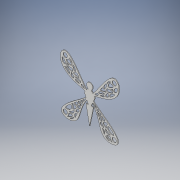
# Autodesk Inventor part: Dragonfly_PCB
Saved by Autodesk Inventor 2019 (Build 230136000, 136)
## iProperties
Created: 2019-03-17
Part Number: Dragonfly_PCB
Material: Generic
Document SubType Name: Modeling
Designer: cutla
Density: 1 g/cm^3
Appearance: Default
Author: cutla
Autodesk Inventor part; units mm, degrees
ref_plane "YZ Plane" through (0, 0, 0) normal (1, 0, 0) x (0, 1, 0)
ref_plane "XZ Plane" through (0, 0, 0) normal (0, 1, 0) x (-1, 0, 0)
ref_plane "XY Plane" through (0, 0, 0) normal (0, 0, 1) x (1, 0, 0)
sketch "Sketch1" plane through (0, 0, 0) normal (0, 0, 1) x (1, 0, 0)
  circle A0 centre (0, 16.1725) radius 5
  line L0 (-50, 50) -> (50, 50) construction
  line L1 (50, 50) -> (50, -50) construction
  line L2 (50, -50) -> (-50, -50) construction
  line L3 (-50, -50) -> (-50, 50) construction
  line L4 (-3.4999, 10.6039) -> (-2.6514, 10.6039)
  line L5 (0, 50) -> (0, -50) construction
  line L6 (-3.5, 10.6039) -> (-8.6386, 3.3725)
  line L7 (-8.6386, 3.3725) -> (-2.5, -10.2779)
  line L8 (2.2173, -10.2779) -> (2.4999, -10.2779)
  line L9 (-6, -11.0793) -> (-0.1613, -40.5057)
  line L10 (-0.1613, -40.5057) -> (6, -11.0793)
  circle A1 centre (-40, 40) radius 23 construction
  circle A2 centre (-40, 40) radius 3.5
  circle A3 centre (-40, 40) radius 6.5 construction
  circle A4 centre (40, 40) radius 23 construction
  circle A5 centre (40, 40) radius 3.5
  circle A6 centre (40, 40) radius 6.5 construction
  line L11 (-50, 0) -> (50, 0) construction
  circle A7 centre (-40, -40) radius 23 construction
  circle A8 centre (-40, -40) radius 3.5
  circle A9 centre (-40, -40) radius 6.5 construction
  circle A10 centre (40, -40) radius 23 construction
  circle A11 centre (40, -40) radius 6.5 construction
  circle A12 centre (40, -40) radius 3.5
  line L12 (-40, 40) -> (40, -40) construction
  line L13 (40, 40) -> (-40, -40) construction
  spline S0 degree 4 poles (-7.4222, 5.0843) (-12.8668, 9.132) (-70.5582, 8.2428) (-44.5421, 80.9884) (-22.7349, 29.3004) (-5.2813, 8.0972) knots 0 0 0 0 0 0.479158 1 1 1 1 1
  spline S1 degree 4 poles (-6, -2.495) (-20.1858, -15.9699) (-90.0237, -50.8952) (-1.0731, -60.254) (-21.894, -29.1199) (-4.4831, -5.8681) knots 0 0 0 0 0 0.512159 1 1 1 1 1
  line L14 (3.5, 10.6039) -> (8.6386, 3.3726)
  line L15 (8.6386, 3.3725) -> (2.5, -10.2779)
  spline S2 degree 4 poles (7.4222, 5.0843) (12.8668, 9.132) (70.5582, 8.2428) (44.5421, 80.9884) (22.7349, 29.3004) (5.2813, 8.0972) knots 0 0 0 0 0 0.479158 1 1 1 1 1
  spline S3 degree 4 poles (6, -2.495) (20.1858, -15.9699) (90.0237, -50.8952) (1.0731, -60.254) (21.894, -29.1199) (4.4831, -5.8681) knots 0 0 0 0 0 0.512159 1 1 1 1 1
  line L16 (-2.1572, -10.5653) -> (-3.3324, -11.0793)
  line L17 (2.1572, -10.5653) -> (3.3324, -11.0793)
  line L18 (-3.0807, 12.2343) -> (-2.6513, 10.6041)
  line L19 (3.0807, 12.2343) -> (2.6513, 10.6041)
  arc A13 (-3.4999, 10.6039) -> (-3.5, 10.6039) centre (-3.4999, 10.6038) ccw
  arc A14 (-2.6514, 10.6039) -> (-2.6513, 10.6041) centre (-2.6514, 10.604) ccw
  line L20 (2.6514, 10.6039) -> (3.4999, 10.6039)
  arc A15 (2.6513, 10.6041) -> (2.6514, 10.6039) centre (2.6514, 10.604) ccw
  arc A16 (3.5, 10.6039) -> (3.4999, 10.6039) centre (3.4999, 10.6038) ccw
  arc A17 (8.6386, 3.3725) -> (8.6386, 3.3726) centre (8.6385, 3.3725) ccw
  arc A18 (1.5005, -10.2779) -> (1.5004, -10.2781) centre (1.5005, -10.278) ccw
  line L21 (-2.5, -10.2779) -> (-2.2173, -10.2779)
  line L22 (-6, -11.0793) -> (-3.3324, -11.0793)
  line L23 (3.3324, -11.0793) -> (6, -11.0793)
  arc A19 (-3.3324, -11.0793) -> (-3.3324, -11.0793) centre (-3.3324, -11.0792) ccw
  arc A20 (-1.5004, -10.2781) -> (-1.5005, -10.2779) centre (-1.5005, -10.278) ccw
  arc A21 (1.5005, -10.2779) -> (1.5004, -10.2781) centre (1.5005, -10.278) ccw
  arc A22 (2.4999, -10.2779) -> (2.5, -10.2779) centre (2.4999, -10.2778) ccw
  arc A23 (3.3324, -11.0793) -> (3.3324, -11.0793) centre (3.3324, -11.0792) ccw
  line L24 (-3.0807, 12.2343) -> (3.0807, 12.2343)
  arc A24 (-2.1572, -10.5653) -> (-2.2173, -10.2779) centre (-2.2173, -10.4279) ccw
  arc A25 (2.2173, -10.2779) -> (2.1572, -10.5653) centre (2.2173, -10.4279) ccw
  point P0 (0, 0)
  point P1 (-3.5, 10.6039)
  point P2 (3.5, 10.6039)
  point P3 (2.5, -10.2779)
  point P4 (-3.5, 10.6039)
  point P5 (0, 25.4731)
  point P6 (0, 0)
  point P7 (0, 2.9442)
  point P8 (-47.4996, 31.0772)
  point P9 (-44.5962, 44.5962)
  point P10 (-36.5, 45.4772)
  point P11 (-30.415, 12.5972)
  point P12 (-44.5962, -35.4038)
  point P13 (-44.5962, -44.5962)
  point P14 (-32.1189, -47.8681)
  point P15 (-20.478, -41.302)
  point P16 (3.5, 10.6039)
  point P17 (8.6386, 3.3725)
  point P18 (47.4996, 31.0772)
  point P19 (44.5962, 44.5962)
  point P20 (36.5, 45.4772)
  point P21 (30.415, 12.5972)
  point P22 (44.5962, -35.4038)
  point P23 (44.5962, -44.5962)
  point P24 (32.1189, -47.8681)
  point P25 (20.478, -41.302)
  point P26 (0, -11.0793)
  point P27 (0, 0)
  point P28 (-1.5, -10.2779)
  point P29 (-3.3324, -11.0793)
  point P30 (1.5, -10.2779)
  point P31 (-2.6512, 10.6039)
  point P32 (2.6512, 10.6039)
  point P33 (3.3324, -11.0793)
  dimension "d0" = 10
  dimension "d1" = 100
  dimension "d2" = 100
  dimension "d3" = 7
  dimension "d5" = 12
  dimension "d6" = 30
  dimension "d7" = 5
  dimension "d8" = 46
  dimension "d9" = 40
  dimension "d10" = 40
  dimension "d11" = 7
  dimension "d12" = 3
  dimension "d13" = 2
  dimension "d14" = 0.0001
  dimension "d15" = 0.0001
  dimension "d16" = 0.0001
  dimension "d24" = 0.15
  constraints: 50 end point, 38 point on line, 30 point on circle, 26 tangent, 25 centre point, 24 symmetric about line, 9 equal radius, 8 horizontal, 6 midpoint, 4 coincident, 4 vertical alignment, 2 parallel, 2 perpendicular, 1 horizontal alignment, 36 other
  measures "d1" distance of L1.end L2.end
  measures "d2" distance of L0.end L1.end
  measures "d3" distance of point (-3.5, 10.604) point (3.5, 10.604)
  measures "d5" distance of L9.start L10.end
  measures "d6" distance of L9.start L9.end
  measures "d7" distance of L7.end point (2.5, -10.278)
  measures "d8" diameter of A1
  measures "d9" distance from line of L5 A1.centre
  measures "d10" horizontal distance of point (0, 0) A1.centre
  measures "d11" diameter of A2
  measures "d12" radial gap between concentric circles of A2 A3
  measures "d13" distance of point (-1.5, -10.278) point (-3.332, -11.079)
  measures "d14" radius of A13
  measures "d15" radius of A15
  measures "d16" radius of A19
  measures "d24" radius of A24
extrude "Extrusion2" add sketch "Sketch1" along normal blind 1 contours A0 L24 | A23 | A19 | A13 | L24 A0 | A0 L19 L20 L14 L15 L8 A25 L17 L23 L10 L9 L22 L16 A24 L21 L7 L6 L4 L18 | L6 S0 | S2 L14 | L7 S1 | S3 L15 | A18 | A20
sketch "Sketch2" plane through (0, 0, 1) normal (0, 0, 1) x (1, 0, 0)
  circle A0 centre (40, 40) radius 3.5 projected
  circle A1 centre (40, -40) radius 3.5 projected
  circle A2 centre (-40, -40) radius 3.5 projected
  circle A3 centre (-40, 40) radius 3.5 projected
  line L0 (-3.0807, 12.2343) -> (-2.6513, 10.6041) projected
  arc A4 (-2.6514, 10.6039) -> (-2.6513, 10.6041) centre (-2.6514, 10.604) ccw projected
  line L1 (-2.6514, 10.6039) -> (-3.4999, 10.6039) projected
  arc A5 (-3.4999, 10.6039) -> (-3.5, 10.6039) centre (-3.4999, 10.6038) ccw projected
  line L2 (-3.5, 10.6039) -> (-5.2813, 8.0972) projected
  line L3 (-7.4222, 5.0843) -> (-8.6386, 3.3725) projected
  line L4 (-8.6386, 3.3725) -> (-6, -2.495) projected
  line L5 (-4.4831, -5.8681) -> (-2.5, -10.2779) projected
  line L6 (-2.5, -10.2779) -> (-2.2173, -10.2779) projected
  line L7 (-2.1572, -10.5653) -> (-3.3324, -11.0793) projected
  arc A6 (-3.3324, -11.0793) -> (-3.3324, -11.0793) centre (-3.3324, -11.0792) ccw projected
  line L8 (-3.3324, -11.0793) -> (-6, -11.0793) projected
  line L9 (-6, -11.0793) -> (-0.1613, -40.5057) projected
  line L10 (-0.1613, -40.5057) -> (6, -11.0793) projected
  line L11 (6, -11.0793) -> (3.3324, -11.0793) projected
  arc A7 (3.3324, -11.0793) -> (3.3324, -11.0793) centre (3.3324, -11.0792) ccw projected
  line L12 (3.3324, -11.0793) -> (2.1572, -10.5653) projected
  line L13 (2.2173, -10.2779) -> (2.4999, -10.2779) projected
  arc A8 (2.4999, -10.2779) -> (2.5, -10.2779) centre (2.4999, -10.2778) ccw projected
  line L14 (2.5, -10.2779) -> (4.4831, -5.8681) projected
  line L15 (6, -2.495) -> (8.6386, 3.3725) projected
  arc A9 (8.6386, 3.3725) -> (8.6386, 3.3726) centre (8.6385, 3.3725) ccw projected
  line L16 (8.6386, 3.3726) -> (7.4222, 5.0843) projected
  line L17 (5.2813, 8.0972) -> (3.5, 10.6039) projected
  arc A10 (3.5, 10.6039) -> (3.4999, 10.6039) centre (3.4999, 10.6038) ccw projected
  line L18 (3.4999, 10.6039) -> (2.6514, 10.6039) projected
  arc A11 (2.6513, 10.6041) -> (2.6514, 10.6039) centre (2.6514, 10.604) ccw projected
  line L19 (2.6513, 10.6041) -> (3.0807, 12.2343) projected
  arc A12 (3.0807, 12.2343) -> (-3.0807, 12.2343) centre (0, 16.1725) ccw projected
  spline S0 degree 5 poles (-44.3024, 35.4148) (-45.0994, 35.5233) (-45.8132, 34.3852) (-44.5065, 29.4541) (-43.5224, 26.3569) (-36.151, 26.1839) (-40.7739, 33.1916) (-43.3141, 35.2801) (-44.3024, 35.4148) knots 0 0 0 0 0 0 0.267852 0.467852 0.667852 1 1 1 1 1 1
  spline S1 degree 5 poles (-40.9057, 24.138) (-41.3791, 23.8252) (-40.5305, 22.4203) (-34.97, 18.6489) (-32.8952, 14.2131) (-29.9643, 20.7538) (-37.6368, 24.0325) (-40.3884, 24.4797) (-40.9057, 24.138) knots 0 0 0 0 0 0 0.286709 0.486709 0.686709 1 1 1 1 1 1
  spline S2 degree 5 poles (-35.4207, 23.9165) (-33.7431, 23.259) (-30.5035, 22.0511) (-26.908, 20.6903) (-24.0215, 30.7808) (-39.446, 25.8859) (-39.0589, 25.3943) (-36.9204, 24.5043) (-35.4207, 23.9165) knots 0 0 0 0 0 0 0.31679 0.51679 0.71679 1 1 1 1 1 1
  spline S3 degree 5 poles (-38.2164, 33.6068) (-38.4732, 34.7959) (-37.0442, 36.9005) (-30.4365, 38.8601) (-30.2842, 28.8387) (-28.4964, 29.5351) (-35.694, 30.5745) (-37.9609, 32.4241) (-38.2164, 33.6068) knots 0 0 0 0 0 0 0.300806 0.500806 0.700806 1 1 1 1 1 1
  spline S4 degree 5 poles (-37.7279, 30.3885) (-37.4976, 30.6871) (-36.795, 30.6092) (-34.7596, 28.9094) (-31.9567, 29.1222) (-38.1366, 27.3933) (-37.545, 26.8348) (-37.9995, 29.2023) (-37.9352, 30.1199) (-37.7279, 30.3885) knots 0 0 0 0 0 0 0.257793 0.412829 0.612829 0.768046 1 1 1 1 1 1
  spline S5 degree 5 poles (-29.5965, 20.8413) (-30.028, 21.0016) (-30.3312, 20.3769) (-29.4621, 17.0894) (-34.8392, 16.5928) (-21.6573, 10.7431) (-26.8093, 18.2659) (-28.9115, 20.5868) (-29.5965, 20.8413) knots 0 0 0 0 0 0 0.231873 0.431873 0.631873 1 1 1 1 1 1
  spline S6 degree 5 poles (-21.2933, 24.138) (-22.1912, 24.1136) (-24.1767, 23.296) (-28.4063, 20.5075) (-28.5904, 21.6776) (-12.6977, 16.5147) (-18.9526, 20.044) (-19.372, 23.4263) (-20.3779, 24.1629) (-21.2933, 24.138) knots 0 0 0 0 0 0 0.240115 0.403809 0.603809 0.755207 1 1 1 1 1 1
  spline S7 degree 5 poles (-23.6063, 17.5202) (-22.4674, 17.6083) (-19.6677, 17.7476) (-15.5206, 18.27) (-8.8964, 8.6854) (-23.9906, 16.981) (-25.349, 17.3364) (-24.46, 17.4541) (-23.6063, 17.5202) knots 0 0 0 0 0 0 0.342928 0.542928 0.742928 1 1 1 1 1 1
  spline S8 degree 5 poles (-22.8794, 14.1718) (-22.1093, 14.3621) (-20.5323, 14.072) (-18.6608, 12.0753) (-11.8654, 10.6615) (-24.2751, 11.1259) (-24.4556, 13.2266) (-23.5584, 14.0041) (-22.8794, 14.1718) knots 0 0 0 0 0 0 0.31884 0.51884 0.71884 1 1 1 1 1 1
  spline S9 degree 5 poles (-12.437, 12.2343) (-11.4678, 12.1009) (-9.6497, 10.9625) (-7.7008, 7.3802) (-7.7483, 8.7391) (-15.1459, 8.7266) (-14.7079, 11.7278) (-13.3583, 12.3611) (-12.437, 12.2343) knots 0 0 0 0 0 0 0.307615 0.507615 0.707615 1 1 1 1 1 1
  spline S10 degree 5 poles (-26.7763, 32.7115) (-26.2605, 32.367) (-25.2409, 31.2314) (-23.9711, 29.2562) (-22.0326, 28.1003) (-24.0441, 19.7801) (-28.4582, 31.1538) (-28.0163, 33.138) (-27.2677, 33.0398) (-26.7763, 32.7115) knots 0 0 0 0 0 0 0.235048 0.414891 0.614891 0.776086 1 1 1 1 1 1
  spline S11 degree 5 poles (-33.5613, 39.3254) (-33.0247, 39.4673) (-31.3289, 38.8651) (-27.3729, 34.9291) (-27.8955, 31.1209) (-31.3505, 38.4233) (-33.3068, 37.2083) (-34.1331, 38.6944) (-33.9123, 39.2325) (-33.5613, 39.3254) knots 0 0 0 0 0 0 0.293287 0.471191 0.671191 0.808125 1 1 1 1 1 1
  line L20 (0, 83.4672) -> (0, -77.3956) construction
  line L21 (-100, 0) -> (100, 0) construction
  spline S12 degree 5 poles (-39.2981, -34.2723) (-39.9524, -33.5365) (-39.0724, -31.2196) (-32.5116, -26.1597) (-30.2015, -22.1531) (-26.383, -31.7521) (-35.2925, -35.1565) (-38.6056, -35.0512) (-39.2981, -34.2723) knots 0 0 0 0 0 0 0.291485 0.491485 0.691485 1 1 1 1 1 1
  spline S13 degree 5 poles (-36.5, -44.8815) (-36.4507, -44.5828) (-35.4911, -43.4851) (-32.644, -40.5677) (-38.0691, -38.4909) (-23.0925, -37.7062) (-29.217, -42.1937) (-35.4081, -45.019) (-36.561, -45.2506) (-36.5, -44.8815) knots 0 0 0 0 0 0 0.213907 0.370528 0.570528 0.735669 1 1 1 1 1 1
  spline S14 degree 5 poles (-32.0039, -45.3695) (-31.8744, -45.6106) (-30.4318, -45.569) (-25.6943, -44.229) (-25.7935, -37.9612) (-26.8264, -42.3738) (-31.1459, -44.3025) (-32.1316, -45.1319) (-32.0039, -45.3695) knots 0 0 0 0 0 0 0.302166 0.502166 0.702166 1 1 1 1 1 1
  spline S15 degree 5 poles (-23.7965, -40) (-23.4775, -39.8625) (-22.9484, -38.6253) (-21.9445, -34.3415) (-17.0929, -31.1562) (-25.8468, -34.6171) (-25.1819, -37.6445) (-24.4279, -39.7279) (-24.0223, -40.0974) (-23.7965, -40) knots 0 0 0 0 0 0 0.272758 0.454007 0.654007 0.806897 1 1 1 1 1 1
  spline S16 degree 5 poles (-33.5613, -36.2711) (-33.4269, -36.7872) (-31.3838, -37.6032) (-24.4371, -38.1393) (-25.5572, -25.7037) (-25.9287, -34.0707) (-32.1902, -34.9016) (-33.6909, -35.7733) (-33.5613, -36.2711) knots 0 0 0 0 0 0 0.305417 0.505417 0.705417 1 1 1 1 1 1
  spline S17 degree 5 poles (-29.099, -22.9229) (-29.0937, -23.4948) (-28.0891, -24.8398) (-24.9737, -27.5316) (-32.4079, -32.1747) (-17.9133, -26.873) (-22.652, -22.0668) (-28.0304, -21.7022) (-29.1046, -22.3167) (-29.099, -22.9229) knots 0 0 0 0 0 0 0.229729 0.394709 0.594709 0.756471 1 1 1 1 1 1
  spline S18 degree 5 poles (-22.3856, -29.8406) (-21.7098, -28.8001) (-20.283, -26.4225) (-18.686, -22.6054) (-13.3004, -31.1371) (-23.325, -31.1181) (-23.5991, -31.589) (-22.9093, -30.647) (-22.3856, -29.8406) knots 0 0 0 0 0 0 0.338056 0.538056 0.738056 1 1 1 1 1 1
  spline S19 degree 5 poles (-25.0368, -20.0903) (-24.9262, -19.1243) (-23.0566, -17.2684) (-16.6088, -15.1482) (-21.8108, -18.0869) (-18.3297, -22.5789) (-23.8077, -22.2725) (-25.1397, -20.99) (-25.0368, -20.0903) knots 0 0 0 0 0 0 0.310671 0.510671 0.710671 1 1 1 1 1 1
  spline S20 degree 5 poles (-20.0653, -23.3991) (-20.1731, -22.7136) (-19.3903, -21.1156) (-15.982, -18.0375) (-17.4847, -19.0811) (-15.059, -22.4523) (-14.2695, -23.7016) (-18.6971, -24.7249) (-19.9485, -24.1412) (-20.0653, -23.3991) knots 0 0 0 0 0 0 0.244633 0.392961 0.592961 0.735209 1 1 1 1 1 1
  spline S21 degree 5 poles (-14.9655, -19.8082) (-15.4817, -19.9871) (-16.0939, -19.275) (-15.7797, -15.6875) (-12.5142, -14.9164) (-11.1676, -13.0261) (-13.0637, -17.9918) (-14.3713, -19.6023) (-14.9655, -19.8082) knots 0 0 0 0 0 0 0.278933 0.478933 0.678933 1 1 1 1 1 1
  spline S22 degree 5 poles (-18.6073, -14.8706) (-18.6874, -15.4171) (-18.5034, -16.4284) (-17.5929, -17.9229) (-17.0852, -19.6506) (-16.7442, -14.6538) (-12.8723, -15.347) (-16.1809, -12.8202) (-18.0104, -13.4255) (-18.5213, -14.2838) (-18.6073, -14.8706) knots 0 0 0 0 0 0 0.195722 0.324759 0.489124 0.649281 0.789869 1 1 1 1 1 1
  spline S23 degree 5 poles (-14.8166, -12.0066) (-14.9241, -12.6125) (-14.4296, -13.5435) (-11.7527, -14.1587) (-9.7456, -11.9141) (-12.6682, -11.6578) (-11.7181, -9.6006) (-13.973, -10.5064) (-14.7175, -11.4477) (-14.8166, -12.0066) knots 0 0 0 0 0 0 0.258357 0.41044 0.61044 0.761675 1 1 1 1 1 1
  spline S24 degree 5 poles (-9.9348, -7.5375) (-10.6244, -8.0811) (-11.5814, -8.9066) (-11.9107, -9.696) (-9.5983, -11.7884) (-7.6983, -7.6612) (-4.6953, -3.5354) (-7.2011, -5.498) (-9.0229, -6.8188) (-9.9348, -7.5375) knots 0 0 0 0 0 0 0.209184 0.360069 0.560069 0.723374 1 1 1 1 1 1
  circle A13 centre (40, -40) radius 3.5
  circle A14 centre (40, 40) radius 3.5
  line L22 (7.4222, 5.0843) -> (8.6386, 3.3725)
  line L23 (8.6386, 3.3725) -> (6, -2.495)
  spline S25 degree 5 poles (44.3024, 35.4148) (45.0994, 35.5233) (45.8132, 34.3852) (44.5065, 29.4541) (43.5224, 26.3569) (36.151, 26.1839) (40.7739, 33.1916) (43.3141, 35.2801) (44.3024, 35.4148) knots 0 0 0 0 0 0 0.267852 0.467852 0.667852 1 1 1 1 1 1
  spline S26 degree 5 poles (40.9057, 24.138) (41.3791, 23.8252) (40.5305, 22.4203) (34.97, 18.6489) (32.8952, 14.2131) (29.9643, 20.7538) (37.6368, 24.0325) (40.3884, 24.4797) (40.9057, 24.138) knots 0 0 0 0 0 0 0.286709 0.486709 0.686709 1 1 1 1 1 1
  spline S27 degree 5 poles (35.4207, 23.9165) (33.7431, 23.259) (30.5035, 22.0511) (26.908, 20.6903) (24.0215, 30.7808) (39.446, 25.8859) (39.0589, 25.3943) (36.9204, 24.5043) (35.4207, 23.9165) knots 0 0 0 0 0 0 0.31679 0.51679 0.71679 1 1 1 1 1 1
  spline S28 degree 5 poles (38.2164, 33.6068) (38.4732, 34.7959) (37.0442, 36.9005) (30.4365, 38.8601) (30.2842, 28.8387) (28.4964, 29.5351) (35.694, 30.5745) (37.9609, 32.4241) (38.2164, 33.6068) knots 0 0 0 0 0 0 0.300806 0.500806 0.700806 1 1 1 1 1 1
  spline S29 degree 5 poles (37.7279, 30.3885) (37.4976, 30.6871) (36.795, 30.6092) (34.7596, 28.9094) (31.9567, 29.1222) (38.1366, 27.3933) (37.545, 26.8348) (37.9995, 29.2023) (37.9352, 30.1199) (37.7279, 30.3885) knots 0 0 0 0 0 0 0.257793 0.412829 0.612829 0.768046 1 1 1 1 1 1
  spline S30 degree 5 poles (29.5965, 20.8413) (30.028, 21.0016) (30.3312, 20.3769) (29.4621, 17.0894) (34.8392, 16.5928) (21.6573, 10.7431) (26.8093, 18.2659) (28.9115, 20.5868) (29.5965, 20.8413) knots 0 0 0 0 0 0 0.231873 0.431873 0.631873 1 1 1 1 1 1
  spline S31 degree 5 poles (21.2933, 24.138) (22.1912, 24.1136) (24.1767, 23.296) (28.4063, 20.5075) (28.5904, 21.6776) (12.6977, 16.5147) (18.9526, 20.044) (19.372, 23.4263) (20.3779, 24.1629) (21.2933, 24.138) knots 0 0 0 0 0 0 0.240115 0.403809 0.603809 0.755207 1 1 1 1 1 1
  spline S32 degree 5 poles (23.6063, 17.5202) (22.4674, 17.6083) (19.6677, 17.7476) (15.5206, 18.27) (8.8964, 8.6854) (23.9906, 16.981) (25.349, 17.3364) (24.46, 17.4541) (23.6063, 17.5202) knots 0 0 0 0 0 0 0.342928 0.542928 0.742928 1 1 1 1 1 1
  spline S33 degree 5 poles (22.8794, 14.1718) (22.1093, 14.3621) (20.5323, 14.072) (18.6608, 12.0753) (11.8654, 10.6615) (24.2751, 11.1259) (24.4556, 13.2266) (23.5584, 14.0041) (22.8794, 14.1718) knots 0 0 0 0 0 0 0.31884 0.51884 0.71884 1 1 1 1 1 1
  spline S34 degree 5 poles (12.437, 12.2343) (11.4678, 12.1009) (9.6497, 10.9625) (7.7008, 7.3802) (7.7483, 8.7391) (15.1459, 8.7266) (14.7079, 11.7278) (13.3583, 12.3611) (12.437, 12.2343) knots 0 0 0 0 0 0 0.307615 0.507615 0.707615 1 1 1 1 1 1
  spline S35 degree 5 poles (26.7763, 32.7115) (26.2605, 32.367) (25.2409, 31.2314) (23.9711, 29.2562) (22.0326, 28.1003) (24.0441, 19.7801) (28.4582, 31.1538) (28.0163, 33.138) (27.2677, 33.0398) (26.7763, 32.7115) knots 0 0 0 0 0 0 0.235048 0.414891 0.614891 0.776086 1 1 1 1 1 1
  spline S36 degree 5 poles (33.5613, 39.3254) (33.0247, 39.4673) (31.3289, 38.8651) (27.3729, 34.9291) (27.8955, 31.1209) (31.3505, 38.4233) (33.3068, 37.2083) (34.1331, 38.6944) (33.9123, 39.2325) (33.5613, 39.3254) knots 0 0 0 0 0 0 0.293287 0.471191 0.671191 0.808125 1 1 1 1 1 1
  spline S37 degree 5 poles (39.2981, -34.2723) (39.9524, -33.5365) (39.0724, -31.2196) (32.5116, -26.1597) (30.2015, -22.1531) (26.383, -31.7521) (35.2925, -35.1565) (38.6056, -35.0512) (39.2981, -34.2723) knots 0 0 0 0 0 0 0.291485 0.491485 0.691485 1 1 1 1 1 1
  spline S38 degree 5 poles (36.5, -44.8815) (36.4507, -44.5828) (35.4911, -43.4851) (32.644, -40.5677) (38.0691, -38.4909) (23.0925, -37.7062) (29.217, -42.1937) (35.4081, -45.019) (36.561, -45.2506) (36.5, -44.8815) knots 0 0 0 0 0 0 0.213907 0.370528 0.570528 0.735669 1 1 1 1 1 1
  spline S39 degree 5 poles (32.0039, -45.3695) (31.8744, -45.6106) (30.4318, -45.569) (25.6943, -44.229) (25.7935, -37.9612) (26.8264, -42.3738) (31.1459, -44.3025) (32.1316, -45.1319) (32.0039, -45.3695) knots 0 0 0 0 0 0 0.302166 0.502166 0.702166 1 1 1 1 1 1
  spline S40 degree 5 poles (23.7965, -40) (23.4775, -39.8625) (22.9484, -38.6253) (21.9445, -34.3415) (17.0929, -31.1562) (25.8468, -34.6171) (25.1819, -37.6445) (24.4279, -39.7279) (24.0223, -40.0974) (23.7965, -40) knots 0 0 0 0 0 0 0.272758 0.454007 0.654007 0.806897 1 1 1 1 1 1
  spline S41 degree 5 poles (33.5613, -36.2711) (33.4269, -36.7872) (31.3838, -37.6032) (24.4371, -38.1393) (25.5572, -25.7037) (25.9287, -34.0707) (32.1902, -34.9016) (33.6909, -35.7733) (33.5613, -36.2711) knots 0 0 0 0 0 0 0.305417 0.505417 0.705417 1 1 1 1 1 1
  spline S42 degree 5 poles (29.099, -22.9229) (29.0937, -23.4948) (28.0891, -24.8398) (24.9737, -27.5316) (32.4079, -32.1747) (17.9133, -26.873) (22.652, -22.0668) (28.0304, -21.7022) (29.1046, -22.3167) (29.099, -22.9229) knots 0 0 0 0 0 0 0.229729 0.394709 0.594709 0.756471 1 1 1 1 1 1
  spline S43 degree 5 poles (22.3856, -29.8406) (21.7098, -28.8001) (20.283, -26.4225) (18.686, -22.6054) (13.3004, -31.1371) (23.325, -31.1181) (23.5991, -31.589) (22.9093, -30.647) (22.3856, -29.8406) knots 0 0 0 0 0 0 0.338056 0.538056 0.738056 1 1 1 1 1 1
  spline S44 degree 5 poles (25.0368, -20.0903) (24.9262, -19.1243) (23.0566, -17.2684) (16.6088, -15.1482) (21.8108, -18.0869) (18.3297, -22.5789) (23.8077, -22.2725) (25.1397, -20.99) (25.0368, -20.0903) knots 0 0 0 0 0 0 0.310671 0.510671 0.710671 1 1 1 1 1 1
  spline S45 degree 5 poles (20.0653, -23.3991) (20.1731, -22.7136) (19.3903, -21.1156) (15.982, -18.0375) (17.4847, -19.0811) (15.059, -22.4523) (14.2695, -23.7016) (18.6971, -24.7249) (19.9485, -24.1412) (20.0653, -23.3991) knots 0 0 0 0 0 0 0.244633 0.392961 0.592961 0.735209 1 1 1 1 1 1
  spline S46 degree 5 poles (14.9655, -19.8082) (15.4817, -19.9871) (16.0939, -19.275) (15.7797, -15.6875) (12.5142, -14.9164) (11.1676, -13.0261) (13.0637, -17.9918) (14.3713, -19.6023) (14.9655, -19.8082) knots 0 0 0 0 0 0 0.278933 0.478933 0.678933 1 1 1 1 1 1
  spline S47 degree 5 poles (18.6073, -14.8706) (18.6874, -15.4171) (18.5034, -16.4284) (17.5929, -17.9229) (17.0852, -19.6506) (16.7442, -14.6538) (12.8723, -15.347) (16.1809, -12.8202) (18.0104, -13.4255) (18.5213, -14.2838) (18.6073, -14.8706) knots 0 0 0 0 0 0 0.195722 0.324759 0.489124 0.649281 0.789869 1 1 1 1 1 1
  spline S48 degree 5 poles (14.8166, -12.0066) (14.9241, -12.6125) (14.4296, -13.5435) (11.7527, -14.1587) (9.7456, -11.9141) (12.6682, -11.6578) (11.7181, -9.6006) (13.973, -10.5064) (14.7175, -11.4477) (14.8166, -12.0066) knots 0 0 0 0 0 0 0.258357 0.41044 0.61044 0.761675 1 1 1 1 1 1
  spline S49 degree 5 poles (9.9348, -7.5375) (10.6244, -8.0811) (11.5814, -8.9066) (11.9107, -9.696) (9.5983, -11.7884) (7.6983, -7.6612) (4.6953, -3.5354) (7.2011, -5.498) (9.0229, -6.8188) (9.9348, -7.5375) knots 0 0 0 0 0 0 0.209184 0.360069 0.560069 0.723374 1 1 1 1 1 1
  arc A15 (-2.1572, -10.5653) -> (-2.2173, -10.2779) centre (-2.2173, -10.4279) ccw projected
  arc A16 (2.2173, -10.2779) -> (2.1572, -10.5653) centre (2.2173, -10.4279) ccw projected
  point P0 (0, 0)
  point P1 (-41.9871, 27.337)
  point P2 (-39.2981, 28.2351)
  point P3 (-32.7821, 17.282)
  point P4 (-32.886, 20.2599)
  point P5 (-28.4118, 26.4199)
  point P6 (-38.05, 25.5602)
  point P7 (-29.8725, 30.7513)
  point P8 (-30.7506, 29.9681)
  point P9 (-34.0552, 28.7609)
  point P10 (-37.2394, 27.4904)
  point P11 (-37.7279, 27.8707)
  point P12 (-30.7506, 16.4205)
  point P13 (-26.1651, 14.4554)
  point P14 (-26.7733, 20.9411)
  point P15 (-17.3741, 18.7332)
  point P16 (-18.8868, 21.8416)
  point P17 (-14.7057, 13.5518)
  point P18 (-24.5877, 17.282)
  point P19 (-16.8157, 11.3031)
  point P20 (-23.7965, 12.9109)
  point P21 (-8.7984, 8.3174)
  point P22 (-14.1289, 10.4452)
  point P23 (-23.0702, 26.8364)
  point P24 (-24.3559, 24.4413)
  point P25 (-27.6589, 32.7115)
  point P26 (-28.5896, 33.887)
  point P27 (-32.1095, 37.3323)
  point P28 (-33.8397, 38.5592)
  point P29 (-30.1416, -25.7925)
  point P30 (-30.2921, -31.1917)
  point P31 (-34.173, -39.4621)
  point P32 (-28.4118, -38.9998)
  point P33 (-26.1775, -40.8544)
  point P34 (-28.346, -42.5329)
  point P35 (-20.4407, -32.9214)
  point P36 (-24.5877, -35.7547)
  point P37 (-24.3559, -39.5636)
  point P38 (-25.5893, -31.1917)
  point P39 (-28.5896, -33.4677)
  point P40 (-27.6471, -29.5079)
  point P41 (-22.3856, -26.635)
  point P42 (-25.8718, -22.2774)
  point P43 (-17.7764, -29.2989)
  point P44 (-23.0702, -31.1917)
  point P45 (-19.5453, -18.2788)
  point P46 (-21.0781, -21.7081)
  point P47 (-16.7273, -19.3246)
  point P48 (-15.5805, -21.8156)
  point P49 (-15.8585, -23.6226)
  point P50 (-12.6799, -14.5271)
  point P51 (-12.1295, -14.6083)
  point P52 (-17.2798, -18.186)
  point P53 (-16.1217, -15.93)
  point P54 (-14.7057, -14.576)
  point P55 (-16.7273, -13.4684)
  point P56 (-10.9965, -12.2195)
  point P57 (-11.8515, -11.1877)
  point P58 (-12.6086, -10.3606)
  point P59 (-10.3983, -10.3606)
  point P60 (-7.7301, -8.073)
  point P61 (-6.3178, -5.1393)
  point P62 (-31.7343, -43.0644)
  point P63 (41.9871, 27.337)
  point P64 (39.2981, 28.2351)
  point P65 (32.7821, 17.282)
  point P66 (32.886, 20.2599)
  point P67 (28.4118, 26.4199)
  point P68 (38.05, 25.5602)
  point P69 (29.8725, 30.7513)
  point P70 (30.7506, 29.9681)
  point P71 (34.0552, 28.7609)
  point P72 (37.2394, 27.4904)
  point P73 (37.7279, 27.8707)
  point P74 (30.7506, 16.4205)
  point P75 (26.1651, 14.4554)
  point P76 (26.7733, 20.9411)
  point P77 (17.3741, 18.7332)
  point P78 (18.8868, 21.8416)
  point P79 (14.7057, 13.5518)
  point P80 (24.5877, 17.282)
  point P81 (16.8157, 11.3031)
  point P82 (23.7965, 12.9109)
  point P83 (8.7984, 8.3174)
  point P84 (14.1289, 10.4452)
  point P85 (23.0702, 26.8364)
  point P86 (24.3559, 24.4413)
  point P87 (27.6589, 32.7115)
  point P88 (28.5896, 33.887)
  point P89 (32.1095, 37.3323)
  point P90 (33.8397, 38.5592)
  point P91 (30.1416, -25.7925)
  point P92 (30.2921, -31.1917)
  point P93 (34.173, -39.4621)
  point P94 (28.4118, -38.9998)
  point P95 (26.1775, -40.8544)
  point P96 (28.346, -42.5329)
  point P97 (20.4407, -32.9214)
  point P98 (24.5877, -35.7547)
  point P99 (24.3559, -39.5636)
  point P100 (25.5893, -31.1917)
  point P101 (28.5896, -33.4677)
  point P102 (27.6471, -29.5079)
  point P103 (22.3856, -26.635)
  point P104 (25.8718, -22.2774)
  point P105 (17.7764, -29.2989)
  point P106 (23.0702, -31.1917)
  point P107 (19.5453, -18.2788)
  point P108 (21.0781, -21.7081)
  point P109 (16.7273, -19.3246)
  point P110 (15.5805, -21.8156)
  point P111 (15.8585, -23.6226)
  point P112 (12.6799, -14.5271)
  point P113 (12.1295, -14.6083)
  point P114 (17.2798, -18.186)
  point P115 (16.1217, -15.93)
  point P116 (14.7057, -14.576)
  point P117 (16.7273, -13.4684)
  point P118 (10.9965, -12.2195)
  point P119 (11.8515, -11.1877)
  point P120 (12.6086, -10.3606)
  point P121 (31.7343, -43.0644)
  point P122 (10.3983, -10.3606)
  point P123 (7.7301, -8.073)
  point P124 (6.3178, -5.1393)
  constraints: 115 symmetric about line, 8 end point, 2 centre point, 1 horizontal, 1 vertical, 230 other
extrude "Extrusion3" cut sketch "Sketch2" against normal through all contours S0 | S1 | S2 | S3 | S4 | S5 | S6 | S7 | S8 | S9 | S10 | S11 | S12 | S13 | S14 | S15 | S16 | S17 | S18 | S19 | S20 | S21 | S22 | S23 | S24 | S25 | S26 | S27 | S28 | S29 | S30 | S31 | S32 | S33 | S34 | S35 | S36 | S37 | S38 | S39 | S40 | S41 | S42 | S43 | S44 | S45 | S46 | S47 | S48 | S49
body "Solid2"
